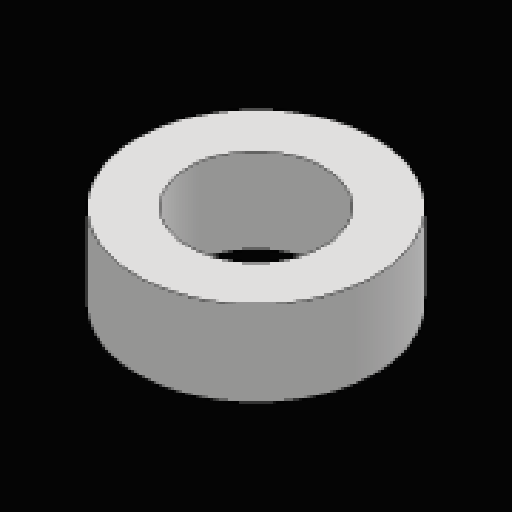
# Autodesk Inventor part: 4x7x2.5mm Bearing
Saved by Autodesk Inventor 2023.2 (Build 272271030, 271C)
## iProperties
Created: 2023-11-12
Part Number: 4x7x2.5mm Bearing
Material: Generic
Document SubType Name: Modeling
Designer: robpl
Density: 1 g/cm^3
Appearance: Default
Author: robpl
Autodesk Inventor part; units mm, degrees
ref_plane "YZ Plane" through (0, 0, 0) normal (1, 0, 0) x (0, 1, 0)
ref_plane "XZ Plane" through (0, 0, 0) normal (0, 1, 0) x (-1, 0, 0)
ref_plane "XY Plane" through (0, 0, 0) normal (0, 0, 1) x (1, 0, 0)
sketch "Sketch1" plane through (0, 0, 0) normal (0, 0, 1) x (1, 0, 0)
  line L0 (0, 0) -> (-3.5, 0)
  line L1 (-3.5, 0) -> (-3.5, -2.5)
  line L2 (-3.5, -2.5) -> (0, -2.5)
  line L3 (0, -2.5) -> (0, 0)
  line L4 (0, 0) -> (-2, 0)
  line L5 (-2, 0) -> (-2, -2.5)
  line L6 (-2, -2.5) -> (0, -2.5)
  line L7 (0, -2.5) -> (0, 0)
  dimension "d0" = 2
  dimension "d1" = 2.5
  dimension "d2" = 3.5
  constraints: 16 end point, 4 parallel, 2 horizontal, 2 perpendicular, 1 point on line
  measures "d0" distance between parallel lines of L3 L5
  measures "d1" distance of L2.end L0.start
  measures "d2" distance of L1.end L2.end
revolve "Revolution1" add sketch "Sketch1" angle 360 about axis through (0, -2.5, 0) along (0, 1, 0) contours L5 L2 L1 L0
body "Solid1"
